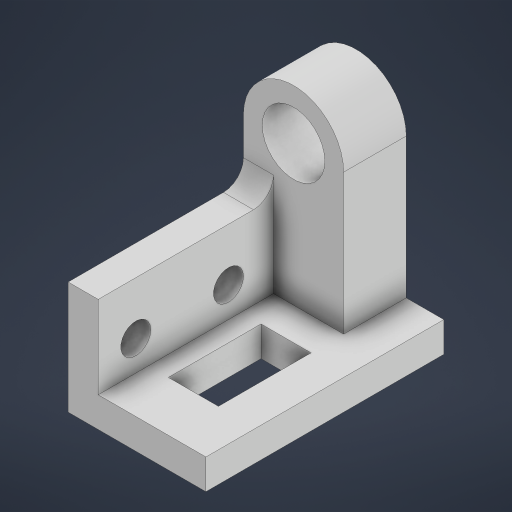
# Autodesk Inventor part: Część5
Saved by Autodesk Inventor 2023 (Build 270158000, 158)
## iProperties
Created: 2023-05-07
Part Number: Część5
Material: Ogólny
Document SubType Name: Modeling
Designer: Adam
Density: 1 g/cm^3
Appearance: Domyślna
Author: Adam
Autodesk Inventor part; units mm, degrees
ref_plane "YZ Plane" through (0, 0, 0) normal (1, 0, 0) x (0, 1, 0)
ref_plane "XZ Plane" through (0, 0, 0) normal (0, 1, 0) x (-1, 0, 0)
ref_plane "XY Plane" through (0, 0, 0) normal (0, 0, 1) x (1, 0, 0)
sketch "Szkic1" plane through (0, 0, 0) normal (0, 1, 0) x (-1, 0, 0)
  line L0 (27.5, 28.9264) -> (-27.5, 28.9264)
  line L1 (-27.5, 28.9264) -> (-27.5, -66.0736)
  line L2 (-27.5, -66.0736) -> (27.5, -66.0736)
  line L3 (27.5, -66.0736) -> (27.5, 28.9264)
  line L4 (-12.5, -28.0736) -> (7.5, -28.0736)
  line L5 (7.5, -28.0736) -> (7.5, 8.9264)
  line L6 (7.5, 8.9264) -> (-12.5, 8.9264)
  line L7 (-12.5, 8.9264) -> (-12.5, -28.0736)
  point P0 (0, 0)
  point P1 (27.5, -18.5736)
  dimension "d0" = 55
  dimension "d1" = 95
  dimension "d3" = 20
  dimension "d4" = 37
  dimension "d5" = 38
  dimension "d6" = 40
  constraints: 16 end point, 4 parallel, 2 horizontal, 2 perpendicular, 1 midpoint
  measures "d0" distance of L2.end L1.end
  measures "d1" distance of L1.end L0.end
  measures "d3" distance between parallel lines of L7 L5
  measures "d4" distance between parallel lines of L4 L6
  measures "d5" distance between parallel lines of L2 L4
  measures "d6" distance from line of point (27.5, -18.574) L7
extrude "Wyciągnięcie proste1" add sketch "Szkic1" along normal blind 12
sketch "Szkic2" plane through (0, 12, 0) normal (0, 1, 0) x (1, 0, 0)
  line L0 (-27.5, 66.0736) -> (-27.5, -28.9264) projected
  line L1 (-27.5, 66.0736) -> (12.5, 66.0736)
  line L2 (12.5, 66.0736) -> (12.5, 41.0736)
  line L3 (12.5, 41.0736) -> (-27.5, 41.0736)
  line L4 (-27.5, 41.0736) -> (-27.5, 66.0736)
  point P0 (0, 0)
  dimension "d9" = 40
  dimension "d10" = 25
  constraints: 8 end point, 2 parallel, 1 horizontal, 1 perpendicular
  measures "d9" distance of L2.end L3.end
  measures "d10" distance of L1.end L2.end
extrude "Wyciągnięcie proste2" add sketch "Szkic2" along normal blind 76
sketch "Szkic3" plane through (0, 12, 0) normal (0, 1, 0) x (1, 0, 0)
  line L0 (-27.5, 66.0736) -> (-27.5, -28.9264) projected
  line L1 (12.5, 41.0736) -> (-27.5, 41.0736) projected
  line L2 (-27.5, -28.9264) -> (-15.5, -28.9264)
  line L3 (-15.5, -28.9264) -> (-15.5, 41.0736)
  line L4 (-15.5, 41.0736) -> (-27.5, 41.0736)
  line L5 (-27.5, 41.0736) -> (-27.5, -28.9264)
  point P0 (0, 0)
  dimension "d13" = 12
  constraints: 8 end point, 2 parallel, 1 horizontal, 1 perpendicular, 1 point on line
  measures "d13" distance of L4.end L3.end
extrude "Wyciągnięcie proste3" add sketch "Szkic3" along normal blind 33
sketch "Szkic4" plane through (-15.5, 12, 28.9264) normal (1, 0, 0) x (0, 0, -1)
  line L0 (0, 0) -> (95, 0) projected
  point P0 (28.9264, -12)
  point P1 (15, 12)
  point P2 (52, 12)
  dimension "d16" = 12
  dimension "d17" = 12
  measures "d16" distance from line of L0 point (15, 12)
  measures "d17" distance from line of L0 point (52, 12)
sketch "Szkic5" plane through (-27.5, 88, -41.0736) normal (0, 0, 1) x (1, 0, 0)
  point P0 (27.5, -88)
  point P1 (20, -20)
hole "Otwór1" at (-15.5, 24, 13.9264) at (-15.5, 24, -23.0736) direction (-1, 0, 0) diameter 12 end through all
hole "Otwór2" at (-7.5, 68, -41.0736) direction (0, 0, -1) diameter 25 end through all
full round fillet "Zaokrąglenie pełne1" first side at (12.5, 62.6667, -49.4069) centre faces at (-14.1667, 88, -57.7402) second side at (-27.5, 44.3333, -57.7402)
fillet "Zaokrąglenie powierzchni1" radius 8 1 edges at (-21.5, 45, -41.0736)
